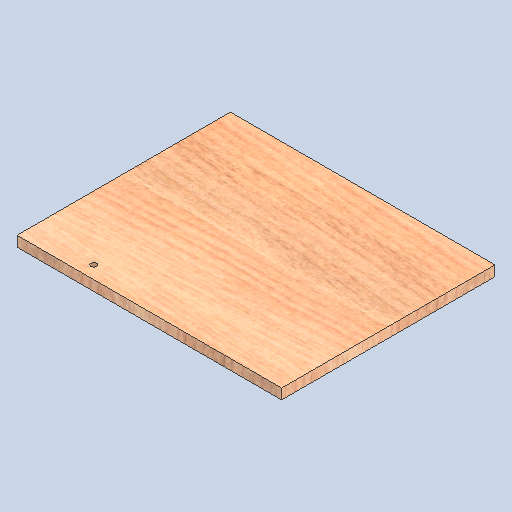
# Autodesk Inventor part: Base_Wood_Plate
Saved by Autodesk Inventor 2023 (Build 270158000, 158)
## iProperties
Created: 2022-10-18
Part Number: Base_Wood_Plate
Material: Wood (Birch)
Document SubType Name: Modeling
Designer: 박동준
Density: 0.55 g/cm^3
Appearance: Birch - Natural Polished
Sheet Metal Rule: Default_mm
품번: 1
Author: 박동준
Autodesk Inventor part; units mm, degrees
ref_plane "YZ Plane" through (0, 0, 0) normal (1, 0, 0) x (0, 1, 0)
ref_plane "XZ Plane" through (0, 0, 0) normal (0, 1, 0) x (-1, 0, 0)
ref_plane "XY Plane" through (0, 0, 0) normal (0, 0, 1) x (1, 0, 0)
sketch "스케치1" plane through (0, 0, 0) normal (0, 1, 0) x (-1, 0, 0)
  line L0 (125, -125) -> (-125, -125)
  line L1 (-125, -125) -> (-125, 125)
  line L2 (-125, 125) -> (125, 125)
  line L3 (125, 125) -> (125, -125)
  point P0 (0, 0)
  point P1 (125, 0)
  point P2 (0, -125)
  dimension "d0" = 250
  dimension "d1" = 250
  constraints: 8 end point, 2 midpoint, 2 parallel, 1 horizontal, 1 horizontal alignment, 1 perpendicular, 1 vertical alignment
  measures "d0" distance of L1.end L2.end
  measures "d1" distance of L0.end L1.end
extrude "돌출1" add sketch "스케치1" along normal mid plane 12
sketch "Sketch2" plane through (0, 6, 0) normal (0, 1, 0) x (1, 0, 0)
  line L0 (-125, -125) -> (-95, -125)
  line L1 (-95, -125) -> (-95, -95)
  line L2 (-95, -95) -> (-125, -95)
  line L3 (-125, -95) -> (-125, -125)
  line L4 (-125, -95) -> (-95, -125)
  line L5 (-95, -95) -> (-125, -125)
  point P0 (0, 0)
  point P1 (-110, -110)
  point P2 (-95, -110)
  point P3 (-110, -95)
  dimension "d5" = 30
  dimension "d6" = 30
  constraints: 12 end point, 2 midpoint, 2 parallel, 1 horizontal, 1 horizontal alignment, 1 perpendicular, 1 vertical alignment
  measures "d5" distance of L2.end L1.end
  measures "d6" distance of L1.end L0.end
sketch "Sketch3" plane through (0, 6, 0) normal (0, 1, 0) x (1, 0, 0)
  line L0 (-125, -125) -> (-125, 125) projected
  line L1 (-125, 125) -> (-185, 125)
  line L2 (-185, 125) -> (-185, -125)
  line L3 (-185, -125) -> (-125, -125)
  line L4 (-125, -125) -> (-125, 125)
  point P0 (0, 0)
  dimension "d7" = 60
  dimension "d8" = 250
  constraints: 8 end point, 2 parallel, 1 horizontal, 1 perpendicular
  measures "d7" distance of L3.end L2.end
  measures "d8" distance of L2.end L1.end
extrude "Extrusion2" add sketch "Sketch3" against normal up to surface (12 mm away)
sketch "Sketch4" plane through (0, -6, 0) normal (0, -1, 0) x (1, 0, 0)
  circle A0 centre (-110, 110) radius 2.5 projected
  point P0 (0, 0)
hole "Hole1" at (-110, -6, 110) direction (0, 1, 0) diameter 6.6 end through all countersink diameter 12.6 countersink angle 90 clearance for "Countersunk Flat Head Screw ISO 2009/7046" size "M6" standard "ISO"
equation "\"d1\" = d0"
equation "\"TransitionRadius\" = BendRadius"
equation "\"BendRadius\" = 0.5"
